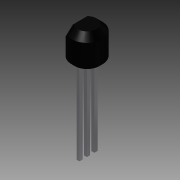
# Autodesk Inventor part: LM35CAZ
Saved by Autodesk Inventor 2014 (Build 180170000, 170)
## iProperties
Created: 2015-11-17
Part Number: LM35CAZ
Material: Generic
Document SubType Name: Modeling
Designer: Owner
Density: 1 g/cm^3
Appearance: Default
Author: Owner
Autodesk Inventor part; units mm, degrees
ref_plane "YZ Plane" through (0, 0, 0) normal (1, 0, 0) x (0, 1, 0)
ref_plane "XZ Plane" through (0, 0, 0) normal (0, 1, 0) x (-1, 0, 0)
ref_plane "XY Plane" through (0, 0, 0) normal (0, 0, 1) x (1, 0, 0)
sketch "Sketch1" plane through (0, 0, 0) normal (0, 1, 0) x (-1, 0, 0)
  circle A0 centre (0, 0) radius 2.6
  line L0 (1.59, 2.0572) -> (1.59, -2.0572)
  dimension "d0" = 5.2
  dimension "d1" = 4.19
  constraints: 2 end point, 2 point on circle, 1 centre point, 1 coincident, 1 vertical
  measures "d0" diameter of A0
extrude "Extrusion1" add sketch "Sketch1" along normal blind 5.2 contours L0 A0 picked at (-1.6247, 0.0943)
sketch "Sketch2" plane through (0, 0, 0) normal (1, 0, 0) x (0, 1, 0)
  line L0 (0, 1.545) -> (-14.2, 1.545)
  line L1 (-14.2, 1.545) -> (-14.2, 0.995)
  line L2 (-14.2, 0.995) -> (0, 0.995)
  line L3 (0, 0.995) -> (0, 1.545)
  line L4 (0, 0.275) -> (-14.2, 0.275)
  line L5 (-14.2, 0.275) -> (-14.2, -0.275)
  line L6 (-14.2, -0.275) -> (0, -0.275)
  line L7 (0, -0.275) -> (0, 0.275)
  line L8 (0, -1.545) -> (-14.2, -1.545)
  line L9 (-14.2, -1.545) -> (-14.2, -0.995)
  line L10 (-14.2, -0.995) -> (0, -0.995)
  line L11 (0, -0.995) -> (0, -1.545)
  line L12 (0, -2.6) -> (0, 2.6) projected
  point P0 (0, 0)
  point P1 (0, 2.0572)
  point P2 (0, -2.0572)
  dimension "d4" = 14.2
  dimension "d5" = 14.2
  dimension "d6" = 14.2
  dimension "d7" = 0
  dimension "d8" = 0
  dimension "d9" = 0.55
  dimension "d10" = 0.55
  dimension "d11" = 0.55
  dimension "d12" = 0.275
  dimension "d13" = 0.995
  dimension "d14" = 0.995
  constraints: 24 end point, 6 parallel, 3 horizontal, 3 perpendicular
  measures "d4" distance of L0.start L0.end
  measures "d5" distance of L4.start L4.end
  measures "d6" distance of L9.end L10.end
  measures "d7" distance between parallel lines of L12 L11
  measures "d8" distance from line of point (0, 0) L7
  measures "d9" distance of L4.end L5.end
  measures "d10" distance of L0.end L1.end
  measures "d11" distance of L8.end L9.end
  measures "d12" distance from line of point (0, 0) L4
  measures "d13" distance from line of L2 point (0, 0)
  measures "d14" distance from line of L10 point (0, 0)
extrude "Extrusion2" add sketch "Sketch2" along normal mid plane 0.5
chamfer "Chamfer1" distance 1 angle 45 1 edges at (2.6, 5.2, 0)
chamfer "Chamfer2" distance 0.5 angle 45 1 edges at (2.6, 0, 0)
chamfer "Chamfer3" distance 0.5 angle 45 3 edges at (-1.59, 4.9218, -0.9998) (-1.59, 4.9218, 0.9998) (-1.59, 5.2, 0)
chamfer "Chamfer4" distance 0.5 angle 45 1 edges at (-1.59, 0, 0)
body "Solid1"
